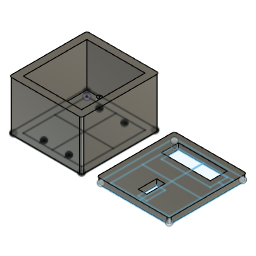
Thick - F3D (Autodesk Fusion 360 design; units mm, degrees)
Autodesk Fusion 360 part; units mm, degrees
note: some values were not read from the file. Set by a fixed rule: which sketch regions a step uses.
sketch "Sketch1" plane through (0, 0, 0) normal (0, 0, 1) x (1, 0, 0)
  line L0 (0, 0) -> (82.55, 0)
  line L1 (82.55, 0) -> (82.55, -90)
  line L2 (82.55, -90) -> (0, -90)
  line L3 (0, -90) -> (0, 0)
  line L4 (89.55, -100) -> (-7, -100)
  line L5 (-10, -97) -> (-10, 7)
  line L6 (-7, 10) -> (89.55, 10)
  line L7 (92.55, 7) -> (92.55, -97)
  arc A0 (-7, 10) -> (-10, 7) centre (-7, 7) ccw
  arc A1 (92.55, 7) -> (89.55, 10) centre (89.55, 7) ccw
  arc A2 (89.55, -100) -> (92.55, -97) centre (89.55, -97) ccw
  arc A3 (-10, -97) -> (-7, -100) centre (-7, -97) ccw
  circle A4 centre (23.475, -5.65) radius 0.943
  circle A5 centre (23.475, -84.35) radius 0.943
  circle A6 centre (59.075, -84.35) radius 0.943
  line L8 (59.075, -84.35) -> (59.075, -90)
  line L9 (23.475, -84.35) -> (23.475, -90)
  circle A7 centre (23.475, -5.65) radius 3
  line L10 (41.275, 0) -> (41.275, -90)
  line L11 (82.55, -45) -> (0, -45)
  circle A8 centre (59.075, -5.65) radius 3
  circle A9 centre (23.475, -84.35) radius 3
  circle A10 centre (59.075, -84.35) radius 3
  line L12 (123.225, 0.9468) -> (205.775, 0.9468)
  arc A11 (215.775, 7.9468) -> (212.775, 10.9468) centre (212.775, 7.9468) ccw
  arc A12 (113.225, -95.883) -> (116.2202, -99.0532) centre (116.2202, -96.0532) ccw
  line L13 (205.775, -44.0532) -> (123.225, -44.0532)
  line L14 (212.775, -99.0532) -> (116.2202, -99.0532)
  line L15 (205.775, 0.9468) -> (205.775, -89.0532)
  line L16 (113.225, -95.883) -> (113.225, 7.9468)
  arc A13 (116.225, 10.9468) -> (113.225, 7.9468) centre (116.225, 7.9468) ccw
  arc A14 (212.775, -99.0532) -> (215.775, -96.0532) centre (212.775, -96.0532) ccw
  line L17 (205.775, -89.0532) -> (123.225, -89.0532)
  line L18 (215.775, 7.9468) -> (215.775, -96.0532)
  line L19 (116.225, 10.9468) -> (212.775, 10.9468)
  line L20 (164.5, 0.9468) -> (164.5, -89.0532)
  line L21 (123.225, -89.0532) -> (123.225, 0.9468)
  line L22 (130, -0.0532) -> (199, -0.0532)
  line L23 (199, -0.0532) -> (199, -24.0532)
  line L24 (199, -24.0532) -> (130, -24.0532)
  line L25 (130, -24.0532) -> (130, -0.0532)
  line L26 (199, -12) -> (205.775, -12)
  circle A15 centre (59.075, -5.65) radius 0.943
  line L27 (158.4929, -59.5532) -> (170.4929, -59.5532)
  line L28 (170.4929, -59.5532) -> (170.4929, -85.5532)
  line L29 (170.4929, -85.5532) -> (158.4929, -85.5532)
  line L30 (158.4929, -85.5532) -> (158.4929, -59.5532)
  point P0 (123.225, 0.9468)
  dimension "d1" = 82.55
  dimension "d2" = 90
  dimension "d4" = 3
  dimension "d5" = 3
  dimension "d6" = 3
  dimension "d7" = 3
  dimension "d8" = 1.886
  dimension "d26" = 6
  dimension "d41" = 82.55
  dimension "d42" = 90
  dimension "d43" = 10
  dimension "d44" = 10
  dimension "d45" = 10
  dimension "d46" = 10
  dimension "d47" = 3
  dimension "d48" = 3
  dimension "d49" = 3
  dimension "d50" = 3
  dimension "d61" = 69
  dimension "d62" = 24
  dimension "d63" = 6.775
  dimension "d64" = 35.6
  dimension "d65" = 78.7
  dimension "d66" = 12
  dimension "d67" = 26
  dimension "d68" = 3.5
  dimension "d69" = 1
  dimension "d78" = 1.886
  dimension "d79" = 1.886
  constraint horizontal L0
  constraint vertical L1
  constraint horizontal L2
  constraint vertical L3
  constraint coincident L0.start L3.end
  constraint tangent L5 A0
  constraint tangent L6 A0
  constraint tangent L6 A1
  constraint tangent L7 A1
  constraint tangent L7 A2
  constraint tangent L4 A2
  constraint tangent L4 A3
  constraint tangent L5 A3
  constraint coincident A6.centre L8.start
  constraint coincident L2 L8.end
  constraint perpendicular L2 L8
  constraint coincident A5.centre L9.start
  constraint coincident L2 L9.end
  constraint perpendicular L2 L9
  constraint concentric A4 A7
  constraint midpoint L0 L10.start
  constraint midpoint L2 L10.end
  constraint midpoint L1 L11.start
  constraint midpoint L3 L11.end
  constraint symmetric A7 L10 A8
  constraint symmetric A7 L11 A9
  constraint symmetric L11 A8 A10
  constraint horizontal L12
  constraint vertical L15
  constraint horizontal L17
  constraint vertical L21
  constraint coincident P0 L12.start
  constraint tangent L16 A13
  constraint tangent A13 L19
  constraint tangent A11 L19
  constraint tangent A11 L18
  constraint tangent A14 L18
  constraint tangent L14 A14
  constraint tangent A12 L14
  constraint midpoint L20.start L12
  constraint midpoint L20.end L17
  constraint midpoint L13.start L15
  constraint midpoint L13.end L21
  constraint horizontal L22
  constraint vertical L23
  constraint horizontal L24
  constraint vertical L25
  constraint coincident L23 L26.start
  constraint coincident L15 L26.end
  constraint perpendicular L15 L26
  constraint symmetric A4 L10 A15
  constraint concentric A5 A9
  constraint concentric A6 A10
  constraint horizontal L27
  constraint vertical L28
  constraint horizontal L29
  constraint vertical L30
  measures "d1" distance of L0.start L0.end
  measures "d2" distance of L0.start L2.end
  measures "d4" radius of A0
  measures "d5" radius of A1
  measures "d6" radius of A2
  measures "d7" radius of A3
  measures "d8" diameter of A4
  measures "d26" diameter of A7
  measures "d41" distance of L12.end P0
  measures "d42" distance of L17.end P0
  measures "d43" distance of L14 L17
  measures "d44" distance of L16 L21
  measures "d45" distance of L12 L19
  measures "d46" distance of L15 L18
  measures "d47" radius of A13
  measures "d48" radius of A11
  measures "d49" radius of A14
  measures "d50" radius of A12
  measures "d61" distance of L23.end L24.end
  measures "d62" distance of L22.start L24.end
  measures "d63" distance of L26.start L26.end
  measures "d64" distance of A4.centre A8.centre
  measures "d65" distance of A4.centre A5.centre
  measures "d66" distance of L27.start L27.end
  measures "d67" distance of L27.start L29.end
  measures "d68" distance of L17 L29
  measures "d69" distance of L12 L22
  measures "d78" diameter of A5
  measures "d79" diameter of A6
extrude "Extrude9" add sketch "Sketch1" along normal blind 8 contours L12 L13 L20 L21 L22 L24 L25 | L12 L15 L20 L22 L23 L26 | L13 L17 L20 L21 L27 L29 L30 | L13 L15 L20 L23 L24 L26 | L13 L15 L17 L20 L27 L28 L29 | A11 A12 L14 L16 A13 A14 L18 L19 makes body 1
sketch "Sketch2" plane through (0, 0, 0) normal (1, 0, 0) x (0, 1, 0)
extrude "Extrude10" add sketch "Sketch1" along normal blind 70 separate body contours L4 L5 L6 L7 A0 A1 A2 A3 makes body 2
extrude "Extrude11" add sketch "Sketch1" along normal blind 14 separate body contours A7 | A8 | A9 | A10 makes body 3 at (62.0601, -5.9487, 9.3333) makes body 4 at (26.2394, -83.1847, 9.3333) makes body 5 at (26.4601, -5.9487, 9.3333) makes body 6 at (61.8394, -83.1847, 9.3333)
extrude "Extrude12" add sketch "Sketch1" along normal blind 8 contours L0 L3 L10 L11 | L0 L1 L10 L11 | L2 L3 L10 L11 | L1 L2 L10 L11 | A4 | A5 | A6 | A15 bodies 2 3 4 5 6
copy_body "Body->Comp2" bodies 2 removing the originals makes body 7 in component "Body"
copy_body "Body->Comp3" bodies 1 removing the originals makes body 8 in component "Lid"
extrude "Extrude6" [suppressed]
extrude "Extrude7" [suppressed]
extrude "Extrude8" [suppressed]
copy_body "Body->Comp1" [suppressed] in component "Component"
component "Body" placed x (1, 0, 0) y (0, 1, 0) z (0, 0, 1) at (0, 0, 0)
component "Lid" placed x (1, 0, 0) y (0, 1, 0) z (0, 0, 1) at (0, 0, 0)
equation "d63 = ( ( 82.55 - 69 ) / 2 ) * 1 mm"
